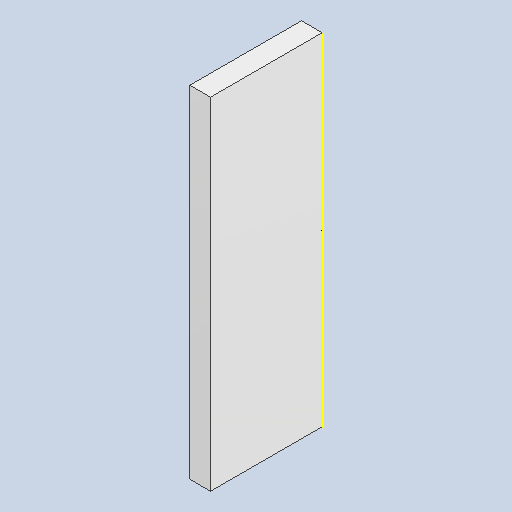
# Autodesk Inventor part: breadboarde
Saved by Autodesk Inventor 2023 (Build 270158000, 158)
## iProperties
Created: 2022-10-02
Part Number: breadboarde
Material: PVC-Piping
Document SubType Name: Modeling
Designer: carso
Density: 1.4 g/cm^3
Appearance: Smooth - White
Author: carso
Autodesk Inventor part; units mm, degrees
ref_plane "YZ Plane" through (0, 0, 0) normal (1, 0, 0) x (0, 1, 0)
ref_plane "XZ Plane" through (0, 0, 0) normal (0, 1, 0) x (-1, 0, 0)
ref_plane "XY Plane" through (0, 0, 0) normal (0, 0, 1) x (1, 0, 0)
sketch "Sketch1" plane through (0, 0, 0) normal (1, 0, 0) x (0, 1, 0)
  line L0 (-82.5, 27) -> (82.5, 27)
  line L1 (82.5, 27) -> (82.5, -27)
  line L2 (82.5, -27) -> (-82.5, -27)
  line L3 (-82.5, -27) -> (-82.5, 27)
  line L4 (-82.5, 27) -> (82.5, -27) construction
  line L5 (82.5, 27) -> (-82.5, -27) construction
  point P0 (0, 0)
  dimension "d0" = 165
  dimension "d1" = 54
  constraints: 12 end point, 2 midpoint, 2 parallel, 1 horizontal, 1 perpendicular
  measures "d0" distance of L1.end L2.end
  measures "d1" distance between parallel lines of L2 L0
extrude "Extrusion1" add sketch "Sketch1" along normal blind 10
sketch "Sketch3" plane through (0, -82.5, -27) normal (0, 0, -1) x (-1, 0, 0)
  line L0 (0, 82.5) -> (-10, 82.5)
  line L1 (-10, 0) -> (-10, 165) projected
  constraints: 2 end point, 1 midpoint
body "Solid1"
